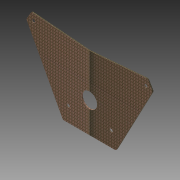
# Autodesk Inventor part: Verboard Middle Plate
Saved by Autodesk Inventor 2015 (Build 190159000, 159)
## iProperties
Created: 2015-10-10
Part Number: Verboard Middle Plate
Material: Veroboard
Document SubType Name: Modeling
Designer: James
Density: 1 g/cm^3
Appearance: Generic
Mass: 5.23229 g
Surface Area: 108.526 cm^2
Volume: 5.23229 cm^3
Author: James
Autodesk Inventor part; units mm, degrees
ref_plane "YZ Plane" through (0, 0, 0) normal (1, 0, 0) x (0, 1, 0)
ref_plane "XZ Plane" through (0, 0, 0) normal (0, 1, 0) x (-1, 0, 0)
ref_plane "XY Plane" through (0, 0, 0) normal (0, 0, 1) x (1, 0, 0)
sketch "Sketch1" plane through (0, 0, 0) normal (0, 1, 0) x (-1, 0, 0)
  line L0 (80.5749, 78.6651) -> (77.2081, 84.4966)
  line L1 (-40.9892, 78.6651) -> (-37.6223, 84.4966)
  line L2 (19.7929, 80.9426) -> (-35.727, 85.4899)
  line L3 (19.7929, 80.9426) -> (75.3128, 85.4899)
  circle A0 centre (-35.159, 78.7632) radius 1.65
  circle A1 centre (74.7448, 78.7632) radius 1.65
  circle A2 centre (-1.1879, 23.9426) radius 1.65
  circle A3 centre (40.7736, 23.9426) radius 1.65
  line L4 (-40.9892, 78.6651) -> (-41.4353, 77.8923)
  line L5 (-41.4699, 75.9547) -> (-6.7517, 10.5409)
  line L6 (-4.9851, 9.4785) -> (44.5709, 9.4785)
  line L7 (80.5749, 78.6651) -> (81.0211, 77.8923)
  line L8 (81.0556, 75.9547) -> (46.3375, 10.5409)
  arc A4 (-35.727, 85.4899) -> (-37.6223, 84.4966) centre (-35.8903, 83.4966) ccw
  arc A5 (77.2081, 84.4966) -> (75.3128, 85.4899) centre (75.476, 83.4966) ccw
  arc A6 (81.0556, 75.9547) -> (81.0211, 77.8923) centre (79.289, 76.8923) ccw
  arc A7 (44.5709, 9.4785) -> (46.3375, 10.5409) centre (44.5709, 11.4785) ccw
  arc A8 (-6.7517, 10.5409) -> (-4.9851, 9.4785) centre (-4.9851, 11.4785) ccw
  arc A9 (-41.4353, 77.8923) -> (-41.4699, 75.9547) centre (-39.7033, 76.8923) ccw
  circle A10 centre (19.7929, 39.09) radius 7.5
  constraints: 18 end point, 12 point on circle, 11 centre point
extrude "Extrusion1" add sketch "Sketch1" along normal blind 1
body "Solid1"
